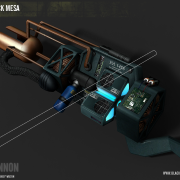
# Autodesk Inventor part: muzzle
Saved by Autodesk Inventor 2020.4 (Build 244396010, 396A)
## iProperties
Created: 2022-09-11
Part Number: muzzle
Material: Generic
Document SubType Name: Modeling
Designer: Val
Density: 1 g/cm^3
Appearance: Default
Author: Val
Autodesk Inventor part; units mm, degrees
ref_plane "YZ Plane" through (0, 0, 0) normal (1, 0, 0) x (0, 1, 0)
ref_plane "XZ Plane" through (0, 0, 0) normal (0, 1, 0) x (-1, 0, 0)
ref_plane "XY Plane" through (0, 0, 0) normal (0, 0, 1) x (1, 0, 0)
sketch "Sketch1" plane through (0, 0, 0) normal (0, 0, 1) x (1, 0, 0)
  circle A0 centre (0, 0) radius 6.35
  dimension "d0" = 12.7
  constraints: 1 centre point, 1 coincident
  measures "d0" diameter of A0
extrude "Extrusion1" add sketch "Sketch1" against normal blind 444.5
body "Solid1"
